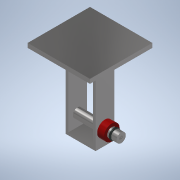
# Autodesk Inventor part: manufacturing link-4
Saved by Autodesk Inventor 2020 (Build 240168000, 168)
## iProperties
Created: 2020-07-27
Part Number: manufacturing link-4
Material: Steel, Mild
Document SubType Name: Modeling
Designer: Vikki
Density: 7.85 g/cm^3
Appearance: Semi-Polished
Mass: 5310.4 g
Surface Area: 692.271 cm^2
Volume: 676.484 cm^3
Author: Vikki
Autodesk Inventor part; units mm, degrees
ref_plane "YZ Plane" through (0, 0, 0) normal (1, 0, 0) x (0, 1, 0)
ref_plane "XZ Plane" through (0, 0, 0) normal (0, 1, 0) x (-1, 0, 0)
ref_plane "XY Plane" through (0, 0, 0) normal (0, 0, 1) x (1, 0, 0)
sketch "Sketch1" plane through (0, 0, 0) normal (0, 1, 0) x (-1, 0, 0)
  line L0 (0, 0) -> (20, 0)
  line L1 (24, 15) -> (20, 15)
  line L2 (20, 15) -> (20, -15)
  line L3 (20, -15) -> (24, -15)
  line L4 (24, -15) -> (24, 15)
  line L5 (0, 0) -> (0, -10) construction
  line L6 (-24, 15) -> (-20, 15)
  line L7 (-20, 15) -> (-20, -15)
  line L8 (-20, -15) -> (-24, -15)
  line L9 (-24, -15) -> (-24, 15)
  point P0 (-20, 0)
  dimension "d0" = 20
  dimension "d1" = 30
  dimension "d2" = 4
  dimension "d3" = 15
  constraints: 20 end point, 5 symmetric about line, 2 horizontal, 2 midpoint, 2 parallel, 1 perpendicular, 1 vertical
  measures "d0" distance of L0.start L0.end
  measures "d1" distance of L1.end L2.end
  measures "d2" distance of L1.start L1.end
  measures "d3" distance from line of L2.end L0
extrude "Extrusion1" add sketch "Sketch1" along normal blind 120
sketch "Sketch2" plane through (-24, 0, -15) normal (-1, 0, 0) x (0, 0, 1)
  circle A0 centre (15, 20) radius 7.5
  line L0 (0, 0) -> (30, 0) projected
  point P0 (15, 0)
  dimension "d6" = 20
  dimension "d7" = 15
  constraints: 1 centre point
  measures "d6" distance from line of L0 A0.centre
  measures "d7" diameter of A0
extrude "Extrusion2" cut sketch "Sketch2" against normal up to surface (48 mm away)
sketch "Sketch3" plane through (0, 0, 0) normal (0, -1, 0) x (1, 0, 0)
  line L0 (24, 15) -> (24, -15) projected
  line L1 (-24, -15) -> (-24, 15) projected
  line L2 (24, -15) -> (-24, -15)
  line L3 (20, 15) -> (24, 15) projected
  line L4 (-24, 15) -> (24, 15)
  point P0 (0, 0)
  constraints: 4 end point, 2 horizontal
extrude "Extrusion3" add sketch "Sketch3" along normal blind 4
sketch "Sketch4" plane through (24, 120, 15) normal (1, 0, 0) x (0, 0, -1)
  circle A0 centre (15, -100) radius 7.5 projected
  circle A1 centre (15, -100) radius 12.5
  point P0 (15, -120)
  dimension "d12" = 25
  constraints: 1 centre point, 1 coincident
  measures "d12" diameter of A1
extrude "Extrusion4" cut sketch "Sketch4" against normal blind 1
sketch "Sketch6" plane through (0, 120, 0) normal (0, 1, 0) x (1, 0, 0)
  line L0 (-50, -50) -> (50, -50)
  line L1 (50, -50) -> (50, 50)
  line L2 (50, 50) -> (-50, 50)
  line L3 (-50, 50) -> (-50, -50)
  line L4 (-50, -50) -> (50, 50) construction
  line L5 (50, -50) -> (-50, 50) construction
  circle A0 centre (-30, 30) radius 12.5
  circle A1 centre (-30, -30) radius 7.5
  circle A2 centre (30, 30) radius 7.5
  circle A3 centre (30, -30) radius 7.5
  circle A4 centre (0, 0) radius 10
  dimension "d15" = 100
  dimension "d16" = 100
  dimension "d17" = 30
  dimension "d18" = 25
  dimension "d20" = 15
  dimension "d21" = 20
  constraints: 12 end point, 5 centre point, 4 point on line, 2 equal radius, 2 horizontal alignment, 2 midpoint, 2 parallel, 1 coincident, 1 horizontal, 1 perpendicular, 1 vertical alignment
  measures "d15" distance of L1.end L2.end
  measures "d16" distance of L0.end L1.end
  measures "d17" horizontal distance of A0.centre point (0, 0)
  measures "d18" diameter of A0
  measures "d20" diameter of A2
  measures "d21" diameter of A4
extrude "Extrusion5" add sketch "Sketch6" along normal blind 3
sketch "Sketch7" plane through (0, 123, 0) normal (0, 1, 0) x (1, 0, 0)
  line L0 (50, 50) -> (-50, 50) projected
  line L1 (-50, 50) -> (-50, -50) projected
  line L2 (-50, -50) -> (50, -50) projected
  line L3 (50, -50) -> (50, 50) projected
  circle A0 centre (-30, 30) radius 12.5 projected
  circle A1 centre (-30, -30) radius 7.5 projected
  circle A2 centre (30, 30) radius 7.5 projected
  circle A3 centre (30, -30) radius 7.5 projected
  circle A4 centre (0, 0) radius 10 projected
extrude "Extrusion6" add sketch "Sketch7" along normal blind 4 contours L3 L2 L1 L0 | A0 | A1 | A2 | A3 | A4
sketch "Sketch8" plane through (24, -4, 15) normal (1, 0, 0) x (0, 0, -1)
  circle A0 centre (15, 24) radius 12.5 projected
  circle A1 centre (15, 24) radius 7.5 projected
  point P0 (15, 4)
extrude "Extrusion7" add sketch "Sketch8" along normal blind 11 and the other way blind 1
sketch "Sketch9" plane through (-24, -4, -15) normal (-1, 0, 0) x (0, 0, 1)
  circle A0 centre (15, 24) radius 7.5 projected
  point P0 (15, 4)
extrude "Extrusion8" add sketch "Sketch9" along normal blind 5 and the other way blind 74
sketch "Sketch10" plane through (50, 20, 0) normal (1, 0, 0) x (0, 0, -1)
  circle A0 centre (0, 0) radius 7.5 projected
  circle A1 centre (0, 0) radius 3
  line L0 (2.2361, -2) -> (-2.2361, -2)
  point P0 (0, -20)
  dimension "d34" = 6
  dimension "d35" = 2
  constraints: 2 end point, 2 point on circle, 1 centre point, 1 coincident
  measures "d34" diameter of A1
  measures "d35" distance from line of A0.centre L0
extrude "Extrusion9" cut sketch "Sketch10" against normal blind 10 contours A1 L0 picked at (0.8351, -0.0457)
ref_plane "Work Plane1" through (38.5, 20, 0) normal (1, 0, 0) x (0, 0, -1)
sketch "Sketch11" plane through (38.5, 20, 0) normal (1, 0, 0) x (0, 0, -1)
  circle A0 centre (0, 0) radius 7.5 projected
  circle A1 centre (0, 0) radius 6
  point P0 (0, -20)
  dimension "d39" = 12
  constraints: 1 centre point, 1 coincident
  measures "d39" diameter of A1
extrude "Extrusion10" cut sketch "Sketch11" along normal blind 3
sketch "Sketch12" plane through (38.5, 20, 0) normal (1, 0, 0) x (0, 0, -1)
  circle A0 centre (0, 0) radius 7.5 projected
  circle A1 centre (0, 0) radius 7.5 projected
  circle A2 centre (0, 0) radius 7.5 projected
  circle A3 centre (0, 0) radius 6.5
  circle A4 centre (0, 0) radius 8.5
  point P0 (0, -20)
  dimension "d42" = 13
  dimension "d43" = 17
  constraints: 2 centre point, 2 coincident
  measures "d42" diameter of A3
  measures "d43" diameter of A4
extrude "Extrusion11" add sketch "Sketch12" along normal blind 2 contours A0 | A4
fillet "Fillet1" radius 4 1 edges at (-24, 20, -7.5)
equation "\"d3\" = 0.5 * d1"
body "Solid1"
